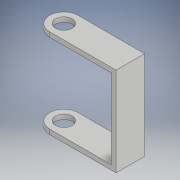
# Autodesk Inventor part: COXA_A
Saved by Autodesk Inventor 2017 (Build 210142000, 142)
## iProperties
Created: 2017-09-18
Part Number: COXA_A
Material: Generic
Document SubType Name: Modeling
Designer: Alexander Miller
Density: 1 g/cm^3
Appearance: Default
Author: Alexander Miller
Autodesk Inventor part; units mm, degrees
ref_plane "YZ Plane" through (0, 0, 0) normal (1, 0, 0) x (0, 1, 0)
ref_plane "XZ Plane" through (0, 0, 0) normal (0, 1, 0) x (-1, 0, 0)
ref_plane "XY Plane" through (0, 0, 0) normal (0, 0, 1) x (1, 0, 0)
sketch "Sketch1" plane through (0, 0, 0) normal (0, 1, 0) x (-1, 0, 0)
  line L0 (18.75, 6) -> (-18.75, 6)
  line L1 (-18.75, 6) -> (-18.75, -6)
  line L2 (-18.75, -6) -> (18.75, -6)
  line L3 (18.75, -6) -> (18.75, 6)
  point P0 (0, 0)
  point P1 (0, 6)
  point P2 (18.75, 0)
  dimension "d0" = 12
  dimension "d1" = 37.5
  constraints: 8 end point, 2 midpoint, 2 parallel, 1 horizontal, 1 horizontal alignment, 1 perpendicular, 1 vertical alignment
  measures "d0" distance of L0.end L1.end
  measures "d1" distance of L1.end L2.end
extrude "Extrusion1" add sketch "Sketch1" along normal blind 2
sketch "Sketch3" plane through (0, 2, 0) normal (0, 1, 0) x (1, 0, 0)
  line L0 (-18.75, 6) -> (-16.75, 6)
  line L1 (-16.75, 6) -> (-16.75, -6)
  line L2 (-16.75, -6) -> (-18.75, -6)
  line L3 (-18.75, -6) -> (-18.75, 6)
  line L4 (16.75, 6) -> (18.75, 6)
  line L5 (18.75, 6) -> (18.75, -6)
  line L6 (18.75, -6) -> (16.75, -6)
  line L7 (16.75, -6) -> (16.75, 6)
  line L8 (18.75, 6) -> (-18.75, 6) projected
  line L9 (-18.75, -6) -> (18.75, -6) projected
  line L10 (-18.75, 6) -> (-18.75, -6) projected
  line L11 (18.75, -6) -> (18.75, 6) projected
  point P0 (0, 0)
  dimension "d8" = 2
  dimension "d9" = 2
  constraints: 16 end point, 6 collinear, 4 parallel, 2 horizontal, 2 perpendicular
  measures "d8" distance between parallel lines of L3 L1
  measures "d9" distance between parallel lines of L5 L7
extrude "Extrusion3" add sketch "Sketch3" along normal blind 32 contours L0 L1 L2 L3 | L4 L5 L6 L7
full round fillet "Fillet3" first side at (-5.5833, 0.6667, 6) centre faces at (17.4167, 34, -2) second side at (5.5833, 0.6667, -6)
full round fillet "Fillet4" first side at (5.5833, 0.6667, -6) centre faces at (-18.0833, 34, -2) second side at (-5.5833, 0.6667, 6)
sketch "Sketch4" plane through (-18.75, 0, -6) normal (-1, 0, 0) x (0, 0, 1)
  circle A0 centre (6, 28) radius 3.5
  arc A1 (12, 28) -> (0, 28) centre (6, 28) ccw projected
  point P0 (6, 0)
  dimension "d12" = 7
  constraints: 1 centre point, 1 concentric
  measures "d12" diameter of A0
extrude "Extrusion4" cut sketch "Sketch4" against normal through all
equation "\"d0\" = servo_B"
equation "\"servo_B\" = 12"
body "Solid1"
